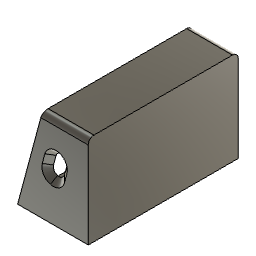
cover (Autodesk Fusion 360 design; units mm, degrees)
Autodesk Fusion 360 part; units mm, degrees
note: some values were not read from the file. Chosen so that the rebuilt part matches the saved one: which pieces of a blend or face edit are solid.
sketch "Sketch1" plane through (0, 0, 0) normal (0, 1, 0) x (1, 0, 0)
  line L0 (0, 0) -> (24, 0)
  line L1 (0, 0) -> (12.941, -48.2963)
  line L2 (0, 0) -> (50, 0) construction
  line L3 (24, 0) -> (36.941, -48.2963)
  line L4 (24, 0) -> (74, 0) construction
  line L5 (12.941, -48.2963) -> (36.941, -48.2963)
  line L6 (36.941, -48.2963) -> (37, 0)
  line L7 (24, 0) -> (37, 0)
  dimension "d1" = 24
  dimension "d2" = 75
  dimension "d3" = 50
  dimension "d4" = 50
  dimension "d5" = 75
  constraint coincident L0.start L1.start
  constraint horizontal L0
  constraint horizontal L2
  constraint horizontal L4
  constraint coincident L4 L6.end
  measures "d1" distance of L0.start L0.end
  measures "d2" angle of L1 L2
  measures "d3" distance of L0.start L1.end
  measures "d4" distance of L0.end L3.end
  measures "d5" angle of L3 L4
extrude "Extrude1" add sketch "Sketch1" along normal blind 78.5
shell "Shell1" thickness 3 removed faces 1 at (4.3137, 26.1667, 16.0988)
sketch "Sketch2" plane through (0, 0, 0) normal (0, -1, 0) x (1, 0, 0)
  line L0 (12.941, 48.2963) -> (0, 0)
  line L1 (0, 0) -> (37, 0)
  line L2 (36.941, 48.2963) -> (12.941, 48.2963)
  line L3 (17.8998, 20.4386) -> (17.8858, 20.4424)
  line L4 (21.5638, 22.5776) -> (22.8982, 27.6553)
  line L5 (20.7731, 31.3156) -> (20.8115, 31.3053)
  line L6 (17.1373, 29.184) -> (15.7785, 24.1128)
  arc A0 (20.8115, 31.3053) -> (17.1373, 29.184) centre (20.0351, 28.4075) ccw
  arc A1 (15.7785, 24.1128) -> (17.8998, 20.4386) centre (18.6763, 23.3364) ccw
  arc A2 (17.8858, 20.4424) -> (21.5638, 22.5776) centre (18.6623, 23.3401) ccw
  arc A3 (22.8982, 27.6553) -> (20.7731, 31.3156) centre (19.9967, 28.4178) ccw
  line L7 (37, 0) -> (36.941, 48.2963)
  point P0 (15.002, 21.2151)
  point P1 (20.7976, 19.6622)
  point P2 (17.9138, 32.0817)
  dimension "d9" = 6
  dimension "d10" = 11.25
  dimension "d11" = 9
  dimension "d12" = 24.375
  dimension "d13" = 3
  constraint coincident P2 L5
  constraint coincident P2 L6
  constraint tangent L5 A0
  constraint tangent L6 A0
  constraint coincident P0 L3
  constraint coincident P0 L6
  constraint tangent L3 A1
  constraint tangent L6 A1
  constraint equal A0 A1
  constraint coincident P1 L3
  constraint coincident P1 L4
  constraint tangent L3 A2
  constraint tangent L4 A2
  constraint equal A0 A2
  constraint tangent L4 A3
  constraint tangent L5 A3
  constraint equal A0 A3
  measures "d9" distance of P0 P1
  measures "d10" distance of P0 P2
  measures "d11" distance of L0 L6
  measures "d12" distance of L0.end L3
  measures "d13" radius of A0
extrude "Extrude2" cut sketch "Sketch2" against normal blind 18 contours L3 L4 L5 L6 A0 A1 A2 A3
chamfer "Chamfer1" distance 3 angle 45 6 edges at (20.1717, 0, 20.7475) (22.231, 0, 25.1165) (22.5961, 0, 29.9154) (16.4579, 0, 26.6484) (16.0764, 0, 21.8395) (18.5265, 0, 31.0006)
fillet "Fillet1" radius 3 2 edges at (24.941, 0, 48.2963) (24.941, 78.5, 48.2963)
equation "d12 = 30 mm - ( 11.25 / 2 ) * 1 mm"
